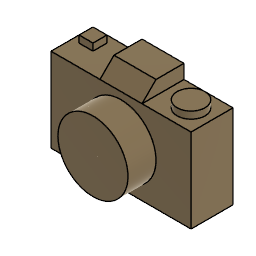
EX-2-1 (Autodesk Fusion 360 design; units mm, degrees)
part number: 2026-04-29-10-15-10-298
Autodesk Fusion 360 part; units mm, degrees
sketch "Sketch1" plane through (0, 0, 0) normal (0, 1, 0) x (1, 0, 0)
  line L0 (0, 0) -> (100, 0)
  line L1 (100, 0) -> (100, -60)
  line L2 (100, -60) -> (0, -60)
  line L3 (0, -60) -> (0, 0)
  dimension "d1" = 100
  dimension "d2" = 60
  constraint horizontal L0
  constraint vertical L1
  constraint horizontal L2
  constraint vertical L3
  constraint coincident L0.start L3.end
  measures "d1" distance of L0.start L0.end
  measures "d2" distance of L0.start L2.end
extrude "Extrude1" add sketch "Sketch1" along normal blind 30
sketch "Sketch2" plane through (0, 0, 0) normal (0, 1, 0) x (1, 0, 0)
  circle A0 centre (50, -30) radius 25
  dimension "d5" = 50
  measures "d5" diameter of A0
extrude "Extrude2" add sketch "Sketch2" against normal blind 20
sketch "Sketch3" plane through (0, 0, 60) normal (0, 0, 1) x (-1, 0, 0)
  line L0 (0, 0) -> (-100, 0)
  line L1 (-100, 0) -> (-100, -30)
  line L2 (-100, -30) -> (0, -30)
  line L3 (0, -30) -> (0, 0)
  line L4 (-5, -25) -> (-15, -25)
  line L5 (-15, -25) -> (-15, -15)
  line L6 (-15, -15) -> (-5, -15)
  line L7 (-5, -15) -> (-5, -25)
  circle A0 centre (-85, -15) radius 10
  dimension "d8" = 20
  dimension "d9" = 15
  dimension "d10" = 10
  dimension "d11" = 10
  dimension "d12" = 15
  dimension "d13" = 15
  dimension "d14" = 15
  constraint horizontal L4
  constraint vertical L5
  constraint horizontal L6
  constraint vertical L7
  measures "d8" diameter of A0
  measures "d9" distance of L3 L5
  measures "d10" distance of L4.start L4.end
  measures "d11" distance of L4.start L6.end
  measures "d12" distance of L2 L6
  measures "d13" distance of L2 A0.centre
  measures "d14" distance of L1 A0.centre
extrude "Extrude3" add sketch "Sketch3" along normal blind 5 contours L4 L5 L6 L7 | A0
sketch "Sketch4" plane through (0, 30, 0) normal (0, 1, 0) x (-1, 0, 0)
  line L0 (0, 60) -> (-100, 60)
  line L1 (-100, 60) -> (-100, 0)
  line L2 (-100, 0) -> (0, 0)
  line L3 (0, 0) -> (0, 60)
  line L4 (-65, 60) -> (-35, 60)
  line L5 (-35, 60) -> (-35, 70)
  line L6 (-35, 70) -> (-65, 70)
  line L7 (-65, 70) -> (-65, 60)
  dimension "d17" = 30
  dimension "d18" = 10
  dimension "d19" = 35
  constraint horizontal L4
  constraint vertical L5
  constraint horizontal L6
  constraint vertical L7
  constraint coincident L0 L4.start
  measures "d17" distance of L5.end L6.end
  measures "d18" distance of L4.end L5.end
  measures "d19" distance of L3 L5
extrude "Extrude4" add sketch "Sketch4" against normal blind 20 contours L0 L4 L5 L6 L7
sketch "Sketch5" plane through (0, 0, 0) normal (1, 0, 0) x (0, 1, 0)
  line L0 (10, 70, 65) -> (10, 60, 65)
  line L1 (0, 60, 100) -> (0, 60, 0)
  line L2 (10, 60, 65) -> (0, 60, 65)
  line L3 (10, 70, 65) -> (0, 60, 65)
  point P0 (30, 70)
  point P1 (30, 60)
  point P2 (10, 70)
  point P3 (10, 60)
  point P4 (10, 70)
  constraint coincident P4 P2
extrude "Extrude5" add sketch "Sketch5" against normal blind 30 contours L0 L2 L3 in plane through (65, 0, 0) normal (1, 0, 0)
